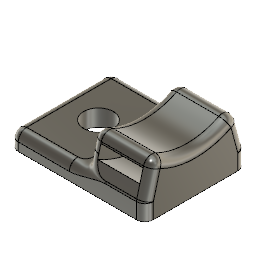
Small_Cable_Tie_Mount (Autodesk Fusion 360 design; units mm, degrees)
Autodesk Fusion 360 part; units mm, degrees
sketch "Sketch1" plane through (0, 0, 0) normal (0, 0, 1) x (1, 0, 0)
  line L0 (0, 0) -> (16, 0)
  line L1 (16, 0) -> (16, 12)
  line L2 (16, 12) -> (0, 12)
  line L3 (0, 12) -> (0, 0)
  circle A0 centre (4.5, 6) radius 1.75
  line L4 (9, 12) -> (9, 0)
  circle A1 centre (4.5, 6) radius 3
  line L5 (0, 0) -> (9, 12) construction
  line L6 (0, 12) -> (9, 0) construction
  dimension "d1" = 16
  dimension "d2" = 12
  dimension "d3" = 3.5
  dimension "d7" = 7
  dimension "d8" = 6
  measures "d3" diameter of A0
  measures "d7" distance of L1 L4
  measures "d8" diameter of A1
extrude "Extrude1" add sketch "Sketch1" along normal blind 2 contours L0 L2 L3 L4 | L0 L1 L2 L4 | A1
extrude "Extrude2" add sketch "Sketch1" along normal blind 10 contours L0 L1 L2 L4
sketch "Sketch2" plane through (16, 0, 0) normal (1, 0, 0) x (0, 1, 0)
  line L0 (0, 0) -> (12, 0)
  line L1 (0, 2) -> (2.1436, 10)
  line L2 (6, 0) -> (6, 10.4384) construction
  line L3 (12, 2) -> (9.8564, 10)
  arc A0 (0.4019, 3.5) -> (11.5981, 3.5) centre (6, 13.1962) ccw
  line L4 (0, 0) -> (12, 0)
  arc A1 (0.7902, 4.9489) -> (11.2098, 4.9489) centre (6, 13.1962) ccw
  arc A2 (1.1784, 6.3978) -> (10.8216, 6.3978) centre (6, 13.1962) ccw
  line L5 (12, 0) -> (12, 10)
  line L6 (0, 10) -> (0, 0)
  line L7 (0, 10) -> (12, 10)
  dimension "d12" = 3.5
  dimension "d13" = 3.5
  dimension "d14" = 1.5
  dimension "d15" = 1.5
  dimension "d27" = 2
  dimension "d28" = 15
  measures "d12" distance of L4
  measures "d13" distance of L4
  measures "d27" distance of L0.start
  measures "d28" angle of L1 L6
extrude "Extrude3" cut sketch "Sketch2" against normal up to surface (16 mm away) contours L1 L6 L7 | L3 L5 L7 | L1 L3 A2 L7
extrude "Extrude4" cut sketch "Sketch2" against normal blind 5 from surface at -1 contours L1 L3 A0 A1
fillet "Fillet5" radius 1 14 edges at (16, 0.5892, 4.1989) (9, 0.5892, 4.1989) (16, 11.4108, 4.1989) (9, 11.4108, 4.1989) (4.5, 12, 2) (9, 6, 2) (0, 6, 2) (0, 12, 1) (4.5, 0, 2) (0, 0, 1) (16, 0, 1) (16, 12, 1) (12.5, 0, 2) (12.5, 12, 2) 1 faces at (13.6667, 5.8096, 4.8637)
